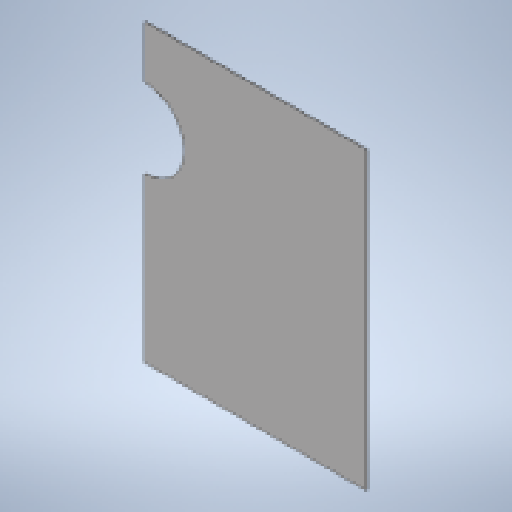
# Autodesk Inventor part: GBK-RK-0017 long wall 3
Saved by Autodesk Inventor 2026.2 (Build 302298000, 298)
## iProperties
Created: 2026-09-14
Part Number: GBK-RK-0017 long wall 3
Material: Generic
Document SubType Name: Sheet Metal
Designer: admin
Density: 1 g/cm^3
Sheet Metal Rule: Default_mm
Appearance: Default
Flat Pattern Width: 120 cm
Flat Pattern Length: 160 cm
Flat Pattern Area: 19200 cm^2
Sheet Metal Width: 1200,000 mm
Sheet Metal Length: 1600,000 mm
Sheet Metal Area: 1920000,000 mm^2
Author: admin
Autodesk Inventor part; units mm, degrees
note: some values were not read from the file. Chosen so that the rebuilt part matches the saved one: flange form of "Plate1".
ref_plane "YZ Plane" through (0, 0, 0) normal (1, 0, 0) x (0, 1, 0)
ref_plane "XZ Plane" through (0, 0, 0) normal (0, 1, 0) x (-1, 0, 0)
ref_plane "XY Plane" through (0, 0, 0) normal (0, 0, 1) x (1, 0, 0)
sketch "Sketch1" plane through (0, 0, 0) normal (1, 0, 0) x (0, 1, 0)
  line L0 (1620, 0) -> (70, 0)
  line L1 (70, 0) -> (20, 0)
  line L2 (20, 0) -> (0, 0)
  dimension "d0" = 180
  dimension "d1" = 50
  dimension "d2" = 1620
  dimension "d3" = 20
  measures "d0" angle of L1 L0
  measures "d1" distance of L0.end L1.end
  measures "d2" distance of L0.start L2.end
  measures "d3" distance of L1.end L2.end
contour flange "Contour Flange1" sketch "Sketch1" thickness 3 bend radius 3 width 1200 along (1, 0, 0) mid plane no both sides no wall seen from (0, 845, 0) lies toward (0, 0, 1) curves L0 L1
bend "Bend1"
corner "Corner1"
sketch "Sketch3" plane through (0, 49.7046, 0) normal (0, 0, -1) x (-1, 0, 0)
  line L0 (-1197.5147, 1570.2954) -> (-1197.5147, -29.7046) construction
  line L1 (0, 1570.2954) -> (0, -29.7046)
  line L2 (-1200, 1570.2954) -> (0, 1570.2954) construction
  line L3 (0, 1570.2954) -> (0, -29.7046) projected
  circle A0 centre (0, 1070.2954) radius 213
  line L4 (0, -29.7046) -> (-1200, -29.7046) projected
  point P0 (0, -49.7046)
  point P1 (0, 0)
  point P2 (0, 857.2954)
  point P3 (0, 1283.2954)
  dimension "d25" = 426
  dimension "d26" = 500
  constraints: 2 end point, 1 centre point, 1 point on line
  measures "d25" diameter of A0
  measures "d26" distance from line of A0.centre L2
extrude "Cut1" cut sketch "Sketch3" against normal blind 3 contours L1 A0 picked at (-58.5713, 1129.0628)
sketch "Sketch2" plane through (1197.8787, 20, 0.8787) normal (0.7071068, 0, 0.7071068) x (0, 1, 0)
  line L0 (1600, 0) -> (0, 0)
  line L1 (0, 0) -> (0, -50)
  line L2 (0, -50) -> (1600, -50)
  line L3 (1600, -50) -> (1600, 0)
  constraints: 6 end point, 1 horizontal, 1 perpendicular, 1 vertical
equation "\"d27\" = Thickness"
equation "\"d4\" = Thickness"
equation "\"d5\" = BendReliefWidth"
equation "\"d6\" = BendReliefDepth"
equation "\"d7\" = MinimumRemnant"
equation "\"d8\" = TransitionRadius"
equation "\"d10\" = BendRadius"
equation "\"d12\" = CornerReliefSize"
equation "\"d13\" = GapSize"
equation "\"d14\" = JacobiRadiusSize"
equation "\"BendRadius\" = Thickness"
equation "\"BendReliefWidth\" = Thickness"
equation "\"BendReliefDepth\" = 0.5 * Thickness"
equation "\"CornerReliefSize\" = 4 * Thickness"
equation "\"MinimumRemnant\" = 2 * Thickness"
equation "\"TransitionRadius\" = BendRadius"
equation "\"JacobiRadiusSize\" = BendRadius"
equation "\"GapSize\" = Thickness"
equation "\"Thickness\" = 3"
body "Solid1"
